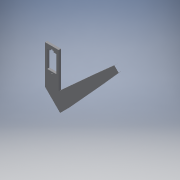
# Autodesk Inventor part: Toe
Saved by Autodesk Inventor 2016 (Build 200138000, 138)
## iProperties
Created: 2015-10-19
Part Number: Toe
Material: Generic
Document SubType Name: Modeling
Designer: powasar16
Density: 1 g/cm^3
Appearance: Default
Author: powasar16
Autodesk Inventor part; units mm, degrees
ref_plane "YZ Plane" through (0, 0, 0) normal (1, 0, 0) x (0, 1, 0)
ref_plane "XZ Plane" through (0, 0, 0) normal (0, 1, 0) x (-1, 0, 0)
ref_plane "XY Plane" through (0, 0, 0) normal (0, 0, 1) x (1, 0, 0)
sketch "Sketch1" plane through (0, 0, 0) normal (0, 0, 1) x (1, 0, 0)
  circle A0 centre (-2.4288, -33.7476) radius 3.75 construction
  line L0 (-6.7056, -28.9306) -> (5.9944, -28.9306)
  line L1 (5.9944, -28.9306) -> (5.9944, -53.0606)
  line L2 (5.9944, -53.0606) -> (-6.7056, -53.0606)
  line L3 (-6.7056, -53.0606) -> (-6.7056, -28.9306)
  line L4 (9.1694, -22.5806) -> (-9.8806, -22.5806)
  line L5 (-9.8806, -22.5806) -> (-9.8806, -117.8306)
  line L6 (9.1694, -71.8398) -> (9.1694, -22.5806)
  line L7 (58.0161, -27.4833) -> (9.1694, -71.8398)
  line L8 (-9.8806, -117.8306) -> (53.7075, -54.2425) construction
  line L9 (115.843, 7.893) -> (102.3726, 21.3634) construction
  line L10 (102.3726, 21.3634) -> (71.3049, -9.7044) construction
  line L11 (5.9944, -38.1) -> (9.1694, -38.1) construction
  line L12 (-6.7056, -38.1) -> (-9.8806, -38.1) construction
  line L13 (53.7075, -54.2425) -> (40.2371, -40.7721) construction
  line L14 (53.7075, -54.2425) -> (84.7753, -23.1747) construction
  line L15 (40.2371, -40.7721) -> (9.1694, -71.8398) construction
  line L16 (84.7753, -23.1747) -> (71.3049, -9.7044) construction
  line L17 (21.9135, -86.0365) -> (9.1694, -71.8398) construction
  arc A1 (107.3117, 16.4242) -> (110.9038, 12.8321) centre (109.1078, 14.6282) ccw construction
  line L18 (84.7753, -23.1747) -> (115.843, 7.893) construction
  line L19 (71.3049, -9.7044) -> (40.2371, -40.7721) construction
  line L20 (69.2414, -38.7086) -> (55.771, -25.2382) construction
  line L21 (21.9135, -86.0365) -> (66.9963, -36.4636)
  line L22 (-9.8806, -117.8306) -> (21.9135, -86.0365)
  line L23 (66.9963, -36.4636) -> (110.9038, 12.8321)
  line L24 (58.0161, -27.4833) -> (107.3117, 16.4242)
  arc A2 (110.9038, 12.8321) -> (107.3117, 16.4242) centre (109.1078, 14.6282) ccw
  line L25 (2.1844, -28.9306) -> (-2.8956, -28.9306)
  line L26 (-2.8956, -28.9306) -> (-2.8956, -27.1526)
  line L27 (-2.8956, -27.1526) -> (2.1844, -27.1526)
  line L28 (2.1844, -27.1526) -> (2.1844, -28.9306)
  line L29 (5.6388, -37.0253) -> (5.6388, -52.2891) projected
  line L30 (5.4388, -52.4891) -> (-6.1612, -52.4891) projected
  dimension "d4" = 5.9944
  dimension "d5" = 5.9944
  dimension "d6" = 12.7
  dimension "d7" = 24.13
  dimension "d8" = 19.05
  dimension "d9" = 95.25
  dimension "d10" = 6.35
  dimension "d12" = 19.05
  dimension "d13" = 177.8
  dimension "d14" = 45
  dimension "d15" = 5.08
  dimension "d16" = 3.175
  dimension "d17" = 3.175
  dimension "d20" = 1.778
  dimension "d21" = 5.08
  dimension "d22" = 3.81
  dimension "d23" = 0.7056
  dimension "d24" = 0.5715
  constraints: 58 end point, 14 perpendicular, 9 point on line, 5 collinear, 5 parallel, 4 midpoint, 4 point on circle, 3 horizontal, 2 centre point
  measures "d6" distance of L0.start L0.end
  measures "d7" distance between parallel lines of L0 L2
  measures "d8" distance between parallel lines of L5 L6
  measures "d9" distance from line of L4 L5.end
  measures "d10" distance between parallel lines of L0 L4
  measures "d12" distance between parallel lines of L10 L8
  measures "d13" distance of L5.end L9.start
  measures "d14" angle of L6 L10
  measures "d15" diameter of A1
  measures "d16" distance from line of L19 L7.start
  measures "d17" distance from line of L14 L21.end
  measures "d20" distance between parallel lines of L0 L27
  measures "d21" distance of L26.end L27.end
  measures "d22" distance between parallel lines of L1 L28
  measures "d24" distance between parallel lines of L2 L30
extrude "Extrusion1" add sketch "Sketch1" along normal blind 3.175
sketch "Sketch2" plane through (0, 0, 3.175) normal (0, 0, 1) x (1, 0, 0)
  arc A0 (-0.8612, -26.1231) -> (0.1388, -26.1231) centre (-0.3612, -26.9891) ccw projected
  arc A1 (0.1388, -55.8551) -> (-0.8612, -55.8551) centre (-0.3612, -54.9891) ccw projected
  circle A2 centre (-0.3612, -54.9891) radius 1
  circle A3 centre (-0.3612, -26.9891) radius 1
  point P0 (0, 0)
  constraints: 2 centre point, 2 coincident, 2 concentric
extrude "Extrusion2" cut sketch "Sketch2" against normal up to next
body "Solid1"
